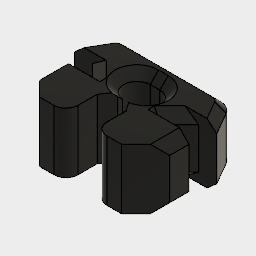
cable_clip_ziptie (Autodesk Fusion 360 design; units mm, degrees)
Autodesk Fusion 360 part; units mm, degrees
note: some values were not read from the file. Set by a fixed rule: which sketch regions a step uses.
sketch "base" plane through (0, 0, 0) normal (0, 0, 1) x (1, 0, 0)
  line L0 (-3.4, 0) -> (-2.2, 0)
  arc A0 (-2.2, 0) -> (-1.2, 1) centre (-2.2, 1) ccw
  line L1 (-1.2, 1) -> (-1.2, 2.5806)
  line L2 (-3.4, 0) -> (-5.4, 2)
  line L3 (-5.4, 3.6) -> (-2.8, 3.6)
  line L4 (-2.8, 3.8) -> (-4.4, 5.4)
  line L5 (-2.2, 0) -> (0, 0) construction
  line L6 (-5.4, 3.6) -> (-5.4, 2)
  arc A1 (-0.3976, 6.1803) -> (-0.5, 3.9803) centre (-0.3976, 5.0779) ccw
  line L7 (-0.3976, 6.1803) -> (0, 6.1803)
  line L8 (-4.4, 5.4) -> (-5.9, 5.4)
  arc A2 (-3.752, 7.8803) -> (-4.826, 7.2602) centre (-3.752, 6.6402) ccw
  line L9 (-3.752, 7.8803) -> (0, 7.8803)
  line L10 (0, 7.8803) -> (0, 0) construction
  line L11 (-2.8, 3.8) -> (-2.8, 3.6)
  line L12 (-5.9, 5.4) -> (-4.826, 7.2602)
  line L13 (-1.2, 2.5806) -> (-0.5, 3.5803)
  line L14 (-0.5, 3.5803) -> (-0.5, 3.9803)
  line L15 (3.752, 7.8803) -> (0, 7.8803)
  arc A3 (4.826, 7.2602) -> (3.752, 7.8803) centre (3.752, 6.6402) ccw
  line L16 (5.9, 5.4) -> (4.826, 7.2602)
  line L17 (4.4, 5.4) -> (5.9, 5.4)
  line L18 (2.8, 3.8) -> (4.4, 5.4)
  line L19 (2.8, 3.8) -> (2.8, 3.6)
  line L20 (5.4, 3.6) -> (2.8, 3.6)
  line L21 (5.4, 3.6) -> (5.4, 2)
  line L22 (3.4, 0) -> (5.4, 2)
  line L23 (3.4, 0) -> (2.2, 0)
  arc A4 (1.2, 1) -> (2.2, 0) centre (2.2, 1) ccw
  line L24 (1.2, 1) -> (1.2, 2.5806)
  line L25 (1.2, 2.5806) -> (0.5, 3.5803)
  line L26 (0.5, 3.5803) -> (0.5, 3.9803)
  arc A5 (0.5, 3.9803) -> (0.3976, 6.1803) centre (0.3976, 5.0779) ccw
  line L27 (0.3976, 6.1803) -> (0, 6.1803)
  dimension "d6" = 4.2
  dimension "d7" = 135
  dimension "d8" = 45
  dimension "d9" = 1
  dimension "d10" = 1.2
  dimension "d27" = 0.2
  dimension "d28" = 2.6
  dimension "d29" = 1.6
  dimension "d31" = 2
  dimension "d32" = 1.8
  dimension "d59" = 1.5
  dimension "d62" = 1.7
  dimension "d64" = 1.5
  dimension "d66" = 0.4
  dimension "d67" = 2.2
  dimension "d68" = 0.5
  dimension "d69" = 1.5
  dimension "d70" = 35
  dimension "d71" = 60
  measures "d6" distance of A0.end L6
  measures "d7" angle of L0 L2
  measures "d8" angle of L3 L4
  measures "d9" radius of A0
  measures "d10" distance of L5.end L1
  measures "d27" distance of L4.start L3.end
  measures "d28" distance of L6 L3.end
  measures "d29" distance of L2.end L3.start
  measures "d31" distance of L0.start L2.end
  measures "d32" distance of L3.start L8
  measures "d59" distance of L4.end L8.end
  measures "d62" distance of L7 L9
  measures "d64" distance of L4 A1
  measures "d66" distance of A1.end L13.end
  measures "d67" distance of A1.end L7
  measures "d68" distance of L10 L14
  measures "d70" angle of L1 L13
  measures "d71" angle of L8 L12
extrude "Extrude1" add sketch "base" along normal blind 5
chamfer "Chamfer1" distance 0.8 angle 45 12 edges at (-5.4, 2.8, 5) (-5.4, 2.8, 0) (-2.8, 3.7, 5) (-3.6, 4.6, 5) (-3.6, 4.6, 0) (-2.8, 3.7, 0) (2.8, 3.7, 5) (3.6, 4.6, 5) (5.4, 2.8, 5) (5.4, 2.8, 0) (2.8, 3.7, 0) (3.6, 4.6, 0)
chamfer "Chamfer3" distance 0.7 angle 45 16 edges at (0, 6.1803, 5) (-1.4988, 5.1292, 0) (0, 6.1803, 0) (-1.4988, 5.1292, 5) (0, 7.8803, 5) (0, 7.8803, 0) (-4.3721, 7.7142, 0) (-4.3721, 7.7142, 5) (-5.363, 6.3301, 5) (-5.363, 6.3301, 0) (1.4988, 5.1292, 0) (1.4988, 5.1292, 5) (5.363, 6.3301, 0) (4.3721, 7.7142, 0) (4.3721, 7.7142, 5) (5.363, 6.3301, 5)
